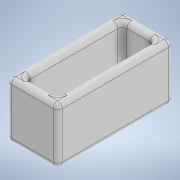
# Autodesk Inventor part: MechanicalPencilLeadCap
Saved by Autodesk Inventor 2020 (Build 240168000, 168)
## iProperties
Created: 2020-09-12
Part Number: MechanicalPencilLeadCap
Material: Generic
Document SubType Name: Modeling
Designer: maple
Density: 1 g/cm^3
Appearance: Default
Author: maple
Autodesk Inventor part; units mm, degrees
ref_plane "YZ Plane" through (0, 0, 0) normal (1, 0, 0) x (0, 1, 0)
ref_plane "XZ Plane" through (0, 0, 0) normal (0, 1, 0) x (-1, 0, 0)
ref_plane "XY Plane" through (0, 0, 0) normal (0, 0, 1) x (1, 0, 0)
sketch "Sketch1" plane through (0, 0, 0) normal (0, 1, 0) x (-1, 0, 0)
  line L0 (0, 0) -> (-7, 0)
  line L1 (-7, 0) -> (-7, -21)
  line L2 (-7, -21) -> (0, -21)
  line L3 (0, -21) -> (0, 0)
  line L4 (0, 0) -> (2, 0)
  line L5 (2, 0) -> (2, 2)
  line L6 (2, 2) -> (0, 2)
  line L7 (0, 2) -> (0, 0)
  line L8 (-7, -21) -> (-9, -21)
  line L9 (-9, -21) -> (-9, -23)
  line L10 (-9, -23) -> (-7, -23)
  line L11 (-7, -23) -> (-7, -21)
  line L12 (-9, -23) -> (2, -23)
  line L13 (2, -23) -> (2, 2)
  line L14 (2, 2) -> (-9, 2)
  line L15 (-9, 2) -> (-9, -23)
  dimension "d0" = 7
  dimension "d1" = 21
  dimension "d2" = 2
  dimension "d3" = 2
  dimension "d4" = 2
  dimension "d5" = 2
  constraints: 32 end point, 8 parallel, 4 horizontal, 4 perpendicular
  measures "d0" distance of L2.end L1.end
  measures "d1" distance of L1.end L0.end
  measures "d2" distance of L6.end L5.end
  measures "d3" distance of L5.end L4.end
  measures "d4" distance of L10.end L9.end
  measures "d5" distance of L9.end L8.end
extrude "Extrusion1" add sketch "Sketch1" along normal blind 2
sketch "Sketch2" plane through (0, 2, 0) normal (0, 1, 0) x (1, 0, 0)
  line L0 (-2, -2) -> (9, -2) projected
  line L1 (-2, -2) -> (0, -2)
  line L2 (0, -2) -> (0, 0)
  line L3 (0, 0) -> (-2, 0)
  line L4 (-2, 0) -> (-2, -2)
  line L5 (9, -2) -> (9, 23) projected
  line L6 (9, 23) -> (7, 23)
  line L7 (7, 23) -> (7, 21)
  line L8 (7, 21) -> (9, 21)
  line L9 (9, 21) -> (9, 23)
  line L10 (0, 0) -> (7, 0)
  line L11 (7, 0) -> (7, 21)
  line L12 (7, 21) -> (0, 21)
  line L13 (0, 21) -> (0, 0)
  line L14 (-2, 23) -> (-2, -2) projected
  line L15 (-2, -2) -> (9, -2)
  line L16 (9, -2) -> (9, 23)
  line L17 (9, 23) -> (-2, 23)
  line L18 (-2, 23) -> (-2, -2)
  dimension "d8" = 2
  dimension "d9" = 2
  dimension "d10" = 2
  dimension "d11" = 2
  constraints: 32 end point, 8 parallel, 4 horizontal, 4 perpendicular
  measures "d8" distance of L3.end L2.end
  measures "d9" distance of L2.end L1.end
  measures "d10" distance of L8.end L7.end
  measures "d11" distance of L7.end L6.end
extrude "Extrusion2" add sketch "Sketch2" along normal blind 10 contours L4 L3 L2 L0 | L2 L10 L11 L8 L5 L0 | L14 L17 L7 L12 L13 L3 | L8 L7 L6 L5
fillet "Fillet1" radius 1 8 edges at (0, 7, -21) (0, 7, 0) (7, 7, 0) (7, 7, -21) (9, 6, 2) (-2, 6, 2) (-2, 6, -23) (9, 6, -23)
fillet "Fillet2" radius 1 32 edges at (0.2929, 2, -0.2929) (3.5, 2, 0) (6.7071, 2, -0.2929) (7, 2, -10.5) (6.7071, 2, -20.7071) (3.5, 2, -21) (0.2929, 2, -20.7071) (0, 2, -10.5) (6.7071, 12, -20.7071) (7, 12, -10.5) (6.7071, 12, -0.2929) (3.5, 12, 0) (0.2929, 12, -0.2929) (0, 12, -10.5) (0.2929, 12, -20.7071) (3.5, 12, -21) (-1.7071, 12, -22.7071) (-2, 12, -10.5) (-1.7071, 12, 1.7071) (3.5, 12, 2) (8.7071, 12, 1.7071) (9, 12, -10.5) (8.7071, 12, -22.7071) (3.5, 12, -23) (8.7071, 0, -22.7071) (3.5, 0, -23) (-1.7071, 0, -22.7071) (-2, 0, -10.5) (-1.7071, 0, 1.7071) (3.5, 0, 2) (8.7071, 0, 1.7071) (9, 0, -10.5)
body "Solid1"
